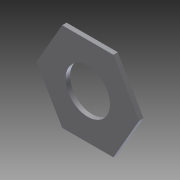
# Autodesk Inventor part: mean machine eye
Saved by Autodesk Inventor 2012 (Build 160160000, 160)
## iProperties
Created: 2013-12-19
Part Number: mean machine eye
Material: Default
Document SubType Name: Modeling
Designer: Bryce
Density: 1 g/cm^3
Author: Bryce
Autodesk Inventor part; units mm, degrees
ref_plane "YZ Plane" through (0, 0, 0) normal (1, 0, 0) x (0, 1, 0)
ref_plane "XZ Plane" through (0, 0, 0) normal (0, 1, 0) x (-1, 0, 0)
ref_plane "XY Plane" through (0, 0, 0) normal (0, 0, 1) x (1, 0, 0)
sketch "Sketch1" plane through (0, 0, 0) normal (0, 0, 1) x (1, 0, 0)
  line L0 (18.3309, 31.75) -> (36.6617, 0)
  line L1 (36.6617, 0) -> (18.3309, -31.75)
  line L2 (18.3309, -31.75) -> (-18.3309, -31.75)
  line L3 (-18.3309, -31.75) -> (-36.6617, 0)
  line L4 (-36.6617, 0) -> (-18.3309, 31.75)
  line L5 (-18.3309, 31.75) -> (18.3309, 31.75)
  circle A0 centre (0, 0) radius 15.875
  dimension "d5" = 63.5
  dimension "d6" = 31.75
  constraints: 12 end point, 2 coincident, 1 centre point, 1 horizontal, 13 other
  measures "d5" distance between parallel lines of L2 L5
  measures "d6" diameter of A0
extrude "Extrusion1" add sketch "Sketch1" along normal blind 3.175
body "Solid1"
